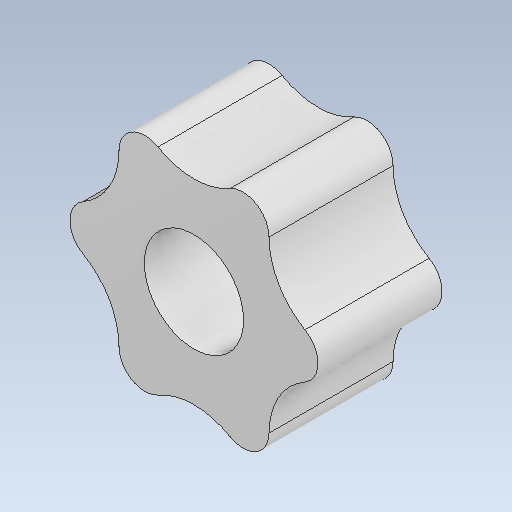
# Autodesk Inventor part: 3ギア接続部
Saved by Autodesk Inventor 2020.4 (Build 244396000, 396)
## iProperties
Created: 2021-05-01
Part Number: 3ギア接続部
Material: アルミニウム 2014-T4
Document SubType Name: Modeling
Designer: happy
Density: 2.8 g/cm^3
Appearance: サテン
Mass: 0.686182 g
Surface Area: 3.17938 cm^2
Volume: 0.245065 cm^3
Author: happy
Autodesk Inventor part; units mm, degrees
ref_plane "YZ Plane" through (0, 0, 0) normal (1, 0, 0) x (0, 1, 0)
ref_plane "XZ Plane" through (0, 0, 0) normal (0, 1, 0) x (-1, 0, 0)
ref_plane "XY Plane" through (0, 0, 0) normal (0, 0, 1) x (1, 0, 0)
sketch "スケッチ1" plane through (0, 0, 0) normal (0, 0, 1) x (1, 0, 0)
  arc A0 (144.025, 105.9095) -> (145.475, 108.4209) centre (142.575, 108.4209) ccw
  arc A1 (145.475, 101.5793) -> (144.025, 104.0908) centre (142.575, 101.5793) ccw
  line L0 (146, 100.67) -> (143.5, 105.0001) construction
  arc A2 (144.025, 105.9095) -> (144.025, 104.0908) centre (144.55, 105.0001) ccw
  line L1 (143.5, 105.0001) -> (146, 109.3303) construction
  circle A3 centre (148.5, 105.0001) radius 5 construction
  arc A4 (149.95, 100.67) -> (147.05, 100.67) centre (148.5, 98.1585) ccw
  line L2 (151, 100.67) -> (146, 100.67) construction
  arc A5 (145.475, 101.5793) -> (147.05, 100.67) centre (146.525, 101.5793) ccw
  arc A6 (149.95, 100.67) -> (151.525, 101.5793) centre (150.475, 101.5793) ccw
  arc A7 (152.975, 104.0908) -> (151.525, 101.5793) centre (154.425, 101.5793) ccw
  line L3 (153.5, 105.0001) -> (151, 100.67) construction
  arc A8 (152.975, 104.0908) -> (152.975, 105.9095) centre (152.45, 105.0001) ccw
  circle A9 centre (148.5, 105.0001) radius 2
  line L4 (151, 109.3303) -> (153.5, 105.0001) construction
  arc A10 (151.525, 108.4209) -> (152.975, 105.9095) centre (154.425, 108.4209) ccw
  arc A11 (151.525, 108.4209) -> (149.95, 109.3303) centre (150.475, 108.4209) ccw
  line L5 (146, 109.3303) -> (151, 109.3303) construction
  arc A12 (147.05, 109.3303) -> (149.95, 109.3303) centre (148.5, 111.8417) ccw
  arc A13 (147.05, 109.3303) -> (145.475, 108.4209) centre (146.525, 108.4209) ccw
  circle A14 centre (148.5, 105.0001) radius 6 construction
  point P0 (0, 0)
  point P1 (146, 100.67)
  point P2 (151, 100.67)
  point P3 (153.5, 105.0001)
  point P4 (145.475, 101.5793)
  point P5 (151.525, 101.5793)
  point P6 (152.975, 104.0908)
  point P7 (152.975, 105.9095)
  point P8 (151.525, 108.4209)
  point P9 (145.475, 108.4209)
  point P10 (144.025, 105.9095)
  point P11 (144.025, 104.0908)
  dimension "d4" = 10
  dimension "d5" = 360
  dimension "d6" = 360
  dimension "d7" = 1.05
  dimension "d8" = 4
  dimension "d9" = 12
  constraints: 30 point on circle, 14 centre point, 12 end point, 4 coincident, 2 point on line, 2 tangent, 1 horizontal alignment, 73 other
  measures "d7" radius of A13
  measures "d8" diameter of A9
  measures "d9" diameter of A14
extrude "押し出し1" add sketch "スケッチ1" along normal blind 5
